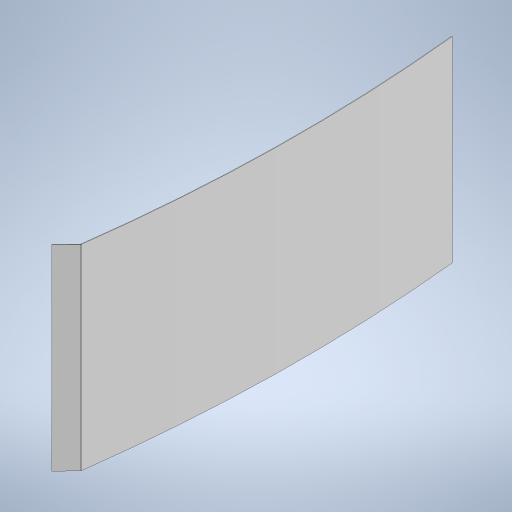
# Autodesk Inventor part: МОО 020 лист борт 1
Saved by Autodesk Inventor 2024.2 (Build 282272000, 272)
## iProperties
Created: 2024-04-28
Part Number: МОО 020 лист борт 1
Material: Generic
Document SubType Name: Sheet Metal
Designer: admin
Density: 1 g/cm^3
Sheet Metal Rule: Default_mm
Appearance: Default
Flat Pattern Width: 100 cm
Flat Pattern Length: 197.467 cm
Flat Pattern Area: 19746.7 cm^2
Sheet Metal Width: 1000,000 mm
Sheet Metal Length: 1974,670 mm
Sheet Metal Area: 1974670,308 mm^2
Author: admin
Autodesk Inventor part; units mm, degrees
note: some values were not read from the file. Chosen so that the rebuilt part matches the saved one: flange form of "Plate1".
ref_plane "YZ Plane" through (0, 0, 0) normal (1, 0, 0) x (0, 1, 0)
ref_plane "XZ Plane" through (0, 0, 0) normal (0, 1, 0) x (-1, 0, 0)
ref_plane "XY Plane" through (0, 0, 0) normal (0, 0, 1) x (1, 0, 0)
sketch "Sketch1" plane through (0, 0, 0) normal (0, 0, 1) x (1, 0, 0)
  line L0 (-750, 0) -> (750, 0) construction
  line L1 (750, 0) -> (750, -2100) construction
  line L2 (750, -2100) -> (110, -2700) construction
  line L3 (108.907697, -2700) -> (-108.907697, -2700) construction
  line L4 (-110, -2700) -> (-750, -2100) construction
  line L5 (-750, -2100) -> (-750, 0) construction
  arc A0 (745.236855, 0.447083) -> (-745.236855, 0.447083) centre (0, -7964.766161) ccw construction
  arc A1 (-750.626493, -4.742884) -> (-776.293231, -222.5) centre (7180.794412, -1050) ccw construction
  arc A2 (-777.58325, -235) -> (-778.853429, -247.5) centre (7180.794412, -1050) ccw construction
  arc A3 (750.128547, -2099.028611) -> (778.853429, -247.5) centre (-7180.794412, -1050) ccw
  arc A4 (777.58325, -235) -> (776.293231, -222.5) centre (-7180.794412, -1050) ccw construction
  line L6 (-777.58325, -235) -> (777.58325, -235) construction
  arc A5 (-749.322934, -2100.70831) -> (-677.569881, -2174.801078) centre (5033.298449, 3427.518345) ccw construction
  line L7 (-750, -2100) -> (750, -2100) construction
  line L8 (-547.172872, -2035.710935) -> (-801.083389, -2306.54882) construction
  arc A6 (-677.569881, -2174.801078) -> (-110.836747, -2699.297556) centre (5033.298449, 3427.518345) ccw construction
  arc A7 (-745.236855, 0.447083) -> (-750.626493, -4.742884) centre (-744.677927, -5.526826) ccw construction
  arc A8 (750.626493, -4.742884) -> (745.236855, 0.447083) centre (744.677927, -5.526826) ccw construction
  arc A9 (-750.128547, -2099.028611) -> (-749.322934, -2100.70831) centre (-747.154451, -2098.635225) ccw construction
  arc A10 (110.836747, -2699.297556) -> (677.569881, -2174.801078) centre (-5033.298449, 3427.518345) ccw construction
  line L9 (553.81945, -2042.800618) -> (794.436811, -2299.459137) construction
  arc A11 (677.569881, -2174.801078) -> (749.322934, -2100.70831) centre (-5033.298449, 3427.518345) ccw
  arc A12 (749.322934, -2100.70831) -> (750.128547, -2099.028611) centre (747.154451, -2098.635225) ccw
  arc A13 (-110.836747, -2699.297556) -> (-108.907697, -2700) centre (-108.907697, -2697) ccw construction
  arc A14 (108.907697, -2700) -> (110.836747, -2699.297556) centre (108.907697, -2697) ccw construction
  line L10 (776.293231, -222.5) -> (-776.293231, -222.5) construction
  line L11 (778.853429, -247.5) -> (-778.853429, -247.5) construction
  arc A15 (778.853429, -247.5) -> (777.58325, -235) centre (-7180.794412, -1050) ccw
  arc A16 (776.293231, -222.5) -> (750.626493, -4.742884) centre (-7180.794412, -1050) ccw construction
  arc A17 (-776.293231, -222.5) -> (-777.58325, -235) centre (7180.794412, -1050) ccw construction
  arc A18 (-778.853429, -247.5) -> (-750.128547, -2099.028611) centre (7180.794412, -1050) ccw construction
  point P0 (0, 0)
  point P1 (0, 0)
  point P2 (0, 0)
  point P3 (0, -2700)
  point P4 (-674.128131, -2171.129877)
  point P5 (674.128131, -2171.129877)
  dimension "d43" = 1500
  dimension "d44" = 2100
  dimension "d45" = 220
  dimension "d46" = 2700
  dimension "d47" = 8000
  dimension "d48" = 8000
  dimension "d49" = 8000
  dimension "d50" = 235
  dimension "d51" = 8000
  dimension "d52" = 104
  dimension "d53" = 6
  dimension "d54" = 3
  dimension "d55" = 8000
  dimension "d56" = 104
  dimension "d57" = 3
  dimension "d67" = 12.5
  dimension "d68" = 12.5
  measures "d43" distance of L0.end L0.start
  measures "d44" distance of L2.start L0.end
  measures "d45" distance of L2.end L4.start
  measures "d46" vertical distance of point (0, -2700) L0.start
  measures "d47" radius of A0
  measures "d48" radius of A1
  measures "d49" radius of A3
  measures "d50" distance between parallel lines of L0 L6
  measures "d51" radius of A5
  measures "d52" distance of L4.end point (-674.128, -2171.13)
  measures "d53" radius of A7
  measures "d54" radius of A9
  measures "d55" radius of A10
  measures "d56" distance of L2.start point (674.128, -2171.13)
  measures "d57" radius of A13
  measures "d67" distance between parallel lines of L6 L10
  measures "d68" distance between parallel lines of L11 L6
contour flange "Contour Flange1" sketch "Sketch1" thickness 3 bend radius 3 width 1000 along (0, 0, 1) mid plane no both sides no wall seen from (713.565816, -2137.870332, 0) lies toward (0.718358, -0.6956736, 0) curves A11 A12 A3 A15
bend "Bend1"
corner "Corner1"
equation "\"d43\" = Бак_ширина_общая"
equation "\"d44\" = Бак_высота_до_конуса"
equation "\"d45\" = Бак_брюхо_ширина_полки"
equation "\"d46\" = Бак_высота_общая"
equation "\"d47\" = Бак_радиус_стенок_общий"
equation "\"d48\" = Бак_радиус_стенок_общий"
equation "\"d49\" = Бак_радиус_стенок_общий"
equation "\"d50\" = Бак_спина_длина_фланцев"
equation "\"d51\" = Бак_радиус_стенок_общий"
equation "\"d52\" = Бак_борт_длина_фланца"
equation "\"d53\" = d65 + d66"
equation "\"d54\" = Thickness"
equation "\"d55\" = Бак_радиус_стенок_общий"
equation "\"d56\" = Бак_борт_длина_фланца"
equation "\"d67\" = Бак_нахлест_фланца"
equation "\"d68\" = Бак_нахлест_фланца"
equation "\"d8\" = Thickness"
equation "\"d9\" = BendReliefWidth"
equation "\"d10\" = BendReliefDepth"
equation "\"d11\" = MinimumRemnant"
equation "\"d12\" = TransitionRadius"
equation "\"d14\" = BendRadius"
equation "\"d16\" = CornerReliefSize"
equation "\"d17\" = GapSize"
equation "\"d18\" = JacobiRadiusSize"
equation "\"BendRadius\" = Thickness"
equation "\"BendReliefWidth\" = Thickness"
equation "\"BendReliefDepth\" = 0.5 * Thickness"
equation "\"CornerReliefSize\" = 4 * Thickness"
equation "\"MinimumRemnant\" = 2 * Thickness"
equation "\"TransitionRadius\" = BendRadius"
equation "\"JacobiRadiusSize\" = BendRadius"
equation "\"GapSize\" = Thickness"
equation "\"d66\" = d65"
equation "\"Бак_ширина_общая\" = 1500"
equation "\"Бак_высота_до_конуса\" = 2100"
equation "\"Бак_брюхо_ширина_полки\" = 220"
equation "\"Бак_радиус_стенок_общий\" = 8000"
equation "\"Бак_спина_длина_фланцев\" = 235"
equation "\"d65\" = 3"
equation "\"Thickness\" = 3"
equation "\"Бак_нахлест_фланца\" = 12.5"
equation "\"Бак_высота_общая\" = 2700"
equation "\"Бак_борт_длина_фланца\" = 104"
body "Solid1"
